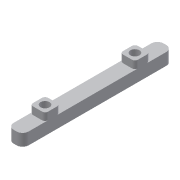
# Autodesk Inventor part: Halter
Saved by Autodesk Inventor 2013 (Build 170138000, 138)
## iProperties
Created: 2013-07-02
Part Number: Halter
Material: Allgemein
Document SubType Name: Modeling
Designer: Harald
Density: 1 g/cm^3
Author: Harald
Autodesk Inventor part; units mm, degrees
ref_plane "YZ Plane" through (0, 0, 0) normal (1, 0, 0) x (0, 1, 0)
ref_plane "XZ Plane" through (0, 0, 0) normal (0, 1, 0) x (-1, 0, 0)
ref_plane "XY Plane" through (0, 0, 0) normal (0, 0, 1) x (1, 0, 0)
sketch "Skizze1" plane through (0, 0, 0) normal (0, 0, 1) x (1, 0, 0)
  line L0 (2, 0) -> (3, 0)
  line L1 (5, 2) -> (5, 48)
  line L2 (3, 50) -> (2, 50)
  line L3 (0, 48) -> (0, 2)
  arc A0 (5, 48) -> (3, 50) centre (3, 48) ccw
  arc A1 (3, 0) -> (5, 2) centre (3, 2) ccw
  arc A2 (0, 2) -> (2, 0) centre (2, 2) ccw
  arc A3 (2, 50) -> (0, 48) centre (2, 48) ccw
  point P0 (0, 0)
  point P1 (5, 50)
  point P2 (5, 0)
  point P3 (0, 50)
  dimension "d0" = 5
  dimension "d1" = 50
  dimension "d2" = 2
  constraints: 8 end point, 8 point on circle, 8 point on line, 8 tangent, 4 centre point, 3 equal radius, 2 parallel, 1 horizontal, 1 perpendicular
  measures "d0" distance of point (0, 50) point (5, 50)
  measures "d1" distance of point (5, 50) point (5, 0)
  measures "d2" radius of A0
extrude "Extrusion1" add sketch "Skizze1" along normal blind 4
sketch "Skizze2" plane through (0, 0, 4) normal (0, 0, 1) x (1, 0, 0)
  line L0 (5, 2) -> (5, 48) projected
  line L1 (3, 50) -> (2, 50) projected
  line L2 (2, 0) -> (3, 0) projected
  line L3 (0, 48) -> (0, 2) projected
  line L4 (1, 42.5) -> (4, 42.5)
  line L5 (5, 41.5) -> (5, 38.5)
  line L6 (4, 37.5) -> (1, 37.5)
  line L7 (0, 38.5) -> (0, 41.5)
  line L8 (1, 12.5) -> (4, 12.5)
  line L9 (5, 11.5) -> (5, 8.5)
  line L10 (4, 7.5) -> (1, 7.5)
  line L11 (0, 8.5) -> (0, 11.5)
  arc A0 (5, 41.5) -> (4, 42.5) centre (4, 41.5) ccw
  arc A1 (4, 37.5) -> (5, 38.5) centre (4, 38.5) ccw
  arc A2 (0, 38.5) -> (1, 37.5) centre (1, 38.5) ccw
  arc A3 (1, 42.5) -> (0, 41.5) centre (1, 41.5) ccw
  arc A4 (5, 11.5) -> (4, 12.5) centre (4, 11.5) ccw
  arc A5 (4, 7.5) -> (5, 8.5) centre (4, 8.5) ccw
  arc A6 (0, 8.5) -> (1, 7.5) centre (1, 8.5) ccw
  arc A7 (1, 12.5) -> (0, 11.5) centre (1, 11.5) ccw
  point P0 (0, 0)
  point P1 (0, 42.5)
  point P2 (5, 37.5)
  point P3 (0, 12.5)
  point P4 (5, 7.5)
  dimension "d12" = 1
  dimension "d13" = 7.5
  dimension "d14" = 5
  dimension "d15" = 5
  dimension "d16" = 7.5
  constraints: 16 end point, 16 point on circle, 16 tangent, 12 point on line, 8 centre point, 7 equal radius, 4 parallel, 2 horizontal, 2 perpendicular
  measures "d12" radius of A0
  measures "d13" distance between parallel lines of L1 L4
  measures "d14" distance between parallel lines of L4 L6
  measures "d15" distance between parallel lines of L10 L8
  measures "d16" distance between parallel lines of L2 L10
extrude "Extrusion2" add sketch "Skizze2" along normal blind 2.5 contours A5 L10 A6 L3 A7 L8 A4 L0 | A1 L6 A2 L3 A3 L4 A0 L0
hole "Bohrung2" at (2.5, 40, 0) direction (0, 0, 1) diameter 3 end through all countersink diameter 4 countersink angle 90
hole "Bohrung3" at (2.5, 10, 0) direction (0, 0, 1) diameter 3 end through all countersink diameter 4 countersink angle 90
equation "\"d15\" = d14"
equation "\"d16\" = d13"
equation "\"d26\" = 0.5 * d0"
equation "\"d27\" = 0.5 * d14"
equation "\"d36\" = 0.5 * d15"
